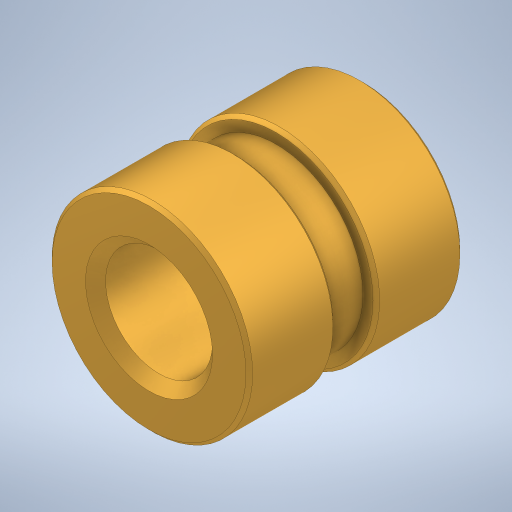
# Autodesk Inventor part: Striped Bushing
Saved by Autodesk Inventor 2023 (Build 270158000, 158)
## iProperties
Created: 2023-02-23
Part Number: Striped Bushing
Material: Brass, Soft Yellow
Document SubType Name: Modeling
Designer: EvanA
Density: 8.47 g/cm^3
Appearance: Brass - Satin
Author: EvanA
Autodesk Inventor part; units mm, degrees
ref_plane "YZ Plane" through (0, 0, 0) normal (1, 0, 0) x (0, 1, 0)
ref_plane "XZ Plane" through (0, 0, 0) normal (0, 1, 0) x (-1, 0, 0)
sketch "Sketch2" plane through (0, 0, 0) normal (0, 0, 1) x (1, 0, 0)
  circle A0 centre (0, 0) radius 4
  circle A1 centre (0, 0) radius 7.5
  dimension "d0" = 8
  dimension "d1" = 15
  constraints: 2 centre point, 2 coincident
  measures "d0" diameter of A0
  measures "d1" diameter of A1
extrude "Extrusion1" add sketch "Sketch2" along normal blind 16
ref_plane "Work Plane1" through (0, 0, 8) normal (0, 0, 1) x (1, 0, 0)
sketch "Sketch3" plane through (0, 0, 8) normal (0, 0, 1) x (1, 0, 0)
  circle A0 centre (0, 0) radius 6.5
  circle A1 centre (0, 0) radius 8
  circle A2 centre (0, 0) radius 4
  dimension "d4" = 13
  dimension "d5" = 16
  dimension "d6" = 8
  constraints: 3 centre point, 3 coincident
  measures "d4" diameter of A0
  measures "d5" diameter of A1
  measures "d6" diameter of A2
extrude "Extrusion2" cut sketch "Sketch3" along normal mid plane 3 contours A1
chamfer "Chamfer1" distance 0.25 angle 45 2 edges at (-7.5, 0, 16) (-7.5, 0, 0)
chamfer "Chamfer2" distance 0.75 angle 45 2 edges at (-4, 0, 16) (-4, 0, 0)
chamfer "Chamfer3" distance 0.25 angle 45 2 edges at (-7.5, 0, 9.5) (-7.5, 0, 6.5)
body "Solid1"
